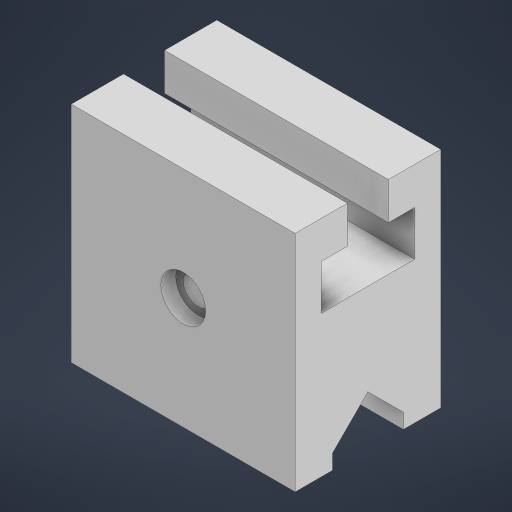
# Autodesk Inventor part: Część3
Saved by Autodesk Inventor 2023 (Build 270158000, 158)
## iProperties
Created: 2023-05-07
Part Number: Część3
Material: Ogólny
Document SubType Name: Modeling
Designer: Adam
Density: 1 g/cm^3
Appearance: Domyślna
Author: Adam
Autodesk Inventor part; units mm, degrees
ref_plane "YZ Plane" through (0, 0, 0) normal (1, 0, 0) x (0, 1, 0)
ref_plane "XZ Plane" through (0, 0, 0) normal (0, 1, 0) x (-1, 0, 0)
ref_plane "XY Plane" through (0, 0, 0) normal (0, 0, 1) x (1, 0, 0)
sketch "Szkic1" plane through (0, 0, 0) normal (1, 0, 0) x (0, 1, 0)
  line L0 (28.1466, 19.5) -> (-31.8534, 19.5)
  line L1 (-31.8534, 19.5) -> (-31.8534, -19.5)
  line L2 (-31.8534, -19.5) -> (28.1466, -19.5)
  line L3 (28.1466, -19.5) -> (28.1466, 19.5)
  line L4 (28.1466, 0) -> (28.1466, 5.5)
  line L5 (28.1466, 5.5) -> (6.1466, 5.5)
  line L6 (6.1466, 5.5) -> (6.1466, 0)
  line L7 (28.1466, -5.5) -> (6.1466, -5.5)
  line L8 (6.1466, -5.5) -> (6.1466, 0)
  line L9 (18.1466, 12.5) -> (6.1466, 12.5)
  line L10 (6.1466, 12.5) -> (6.1466, -12.5)
  line L11 (6.1466, -12.5) -> (18.1466, -12.5)
  line L12 (18.1466, -12.5) -> (18.1466, 12.5)
  line L13 (-31.8534, 9.5) -> (-27.8534, 9.5)
  line L14 (-27.8534, 9.5) -> (-18.3534, 0)
  line L15 (-31.8534, 0) -> (0, 0)
  line L16 (-31.8534, -9.5) -> (-27.8534, -9.5)
  line L17 (-27.8534, -9.5) -> (-18.3534, 0)
  point P0 (12.1466, 0)
  point P1 (6.1466, 2.75)
  point P2 (18.1466, -5.5)
  point P3 (6.1466, -5.5)
  point P4 (18.1466, 5.5)
  dimension "d0" = 60
  dimension "d1" = 39
  dimension "d2" = 22
  dimension "d4" = 12
  dimension "d5" = 25
  dimension "d6" = 135
  dimension "d7" = 10
  dimension "d8" = 4
  dimension "d9" = 9.5
  constraints: 36 end point, 5 parallel, 4 perpendicular, 3 horizontal, 3 midpoint, 3 point on line, 2 symmetric about line, 1 collinear
  measures "d0" distance of L2.end L1.end
  measures "d1" distance of L1.end L0.end
  measures "d2" distance of L5.end L4.end
  measures "d4" distance of L11.end L10.end
  measures "d5" distance of L10.end L9.end
  measures "d6" angle of L13 L14
  measures "d7" distance between parallel lines of L13 L0
  measures "d8" distance of L13.start L13.end
  measures "d9" horizontal distance of L14.end L13.end
extrude "Wyciągnięcie proste1" add sketch "Szkic1" along normal blind 60 contours L3 L5 L12 L9 L10 L6 L8 L11 L7 L2 L1 L16 L17 L14 L13 L0
sketch "Szkic2" plane through (0, -31.8534, 19.5) normal (0, 0, 1) x (1, 0, 0)
  point P0 (0, 31.8534)
  point P1 (30, 30)
hole "Otwór1" at (30, -1.8534, 19.5) direction (0, 0, -1) diameter 8 end through all counterbore diameter 12 counterbore depth 4
